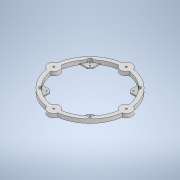
# Autodesk Inventor part: RL_spider_center_bottom_vt
Saved by Autodesk Inventor 2022 (Build 260153000, 153)
## iProperties
Created: 2021-08-09
Part Number: RL_spider_center_bottom_vt
Material: Generic
Document SubType Name: Modeling
Designer: james
Density: 1 g/cm^3
Appearance: Default
Author: james
Autodesk Inventor part; units mm, degrees
ref_plane "YZ Plane" through (0, 0, 0) normal (1, 0, 0) x (0, 1, 0)
ref_plane "XZ Plane" through (0, 0, 0) normal (0, 1, 0) x (-1, 0, 0)
ref_plane "XY Plane" through (0, 0, 0) normal (0, 0, 1) x (1, 0, 0)
sketch "Sketch1" plane through (0, 0, 0) normal (0, 1, 0) x (-1, 0, 0)
  circle A0 centre (0, 0) radius 100
  dimension "d0" = 200
  constraints: 1 centre point, 1 coincident
  measures "d0" diameter of A0
extrude "Extrusion1" add sketch "Sketch1" along normal blind 10
sketch "Sketch15" plane through (0, 10, 0) normal (0, 1, 0) x (1, 0, 0)
  circle A0 centre (0, 0) radius 90
  dimension "d139" = 180
  constraints: 1 centre point, 1 coincident
  measures "d139" diameter of A0
extrude "Extrusion13" cut sketch "Sketch15" against normal blind 20
sketch "Sketch19" plane through (0, 0, 0) normal (0, -1, 0) x (1, 0, 0)
  arc A0 (90, 0) -> (90, 0) centre (0, 0) ccw
  line L0 (49.497475, -56.568542) -> (56.568542, -49.497475)
  line L1 (0, 0) -> (53.033009, -53.033009)
  line L2 (0, 0) -> (1.922714, 0)
  line L3 (53.033009, -53.033009) -> (70.710678, -70.710678)
  circle A1 centre (0, 0) radius 100
  line L4 (49.497475, -56.568542) -> (49.497475, -75.166482)
  line L5 (56.568542, -49.497475) -> (75.166482, -49.497475)
  circle A2 centre (63.993164, -63.993164) radius 1.75
  circle A3 centre (56.922096, -56.922096) radius 1.75
  circle A4 centre (0, 0) radius 90
  point P0 (62.4461, -64.811146)
  point P1 (64.811146, -62.4461)
  dimension "d162" = 45
  dimension "d164" = 25
  dimension "d165" = 135
  dimension "d166" = 135
  dimension "d167" = 3.5
  dimension "d168" = 3.5
  dimension "d169" = 9.5
  dimension "d170" = 19.5
  dimension "d181" = 10
  constraints: 12 end point, 3 centre point, 2 point on circle, 2 point on line, 1 coincident, 1 horizontal, 1 midpoint, 1 perpendicular, 2 other
  measures "d162" angle of L1 L2
  measures "d164" distance from line of L3.end L0
  measures "d165" angle of L5 L0
  measures "d166" angle of L4 L0
  measures "d167" diameter of A3
  measures "d168" diameter of A2
  measures "d169" distance of L3.end A2.centre
  measures "d170" distance of L3.end A3.centre
  measures "d181" distance of L0.start L0.end
extrude "Extrusion16" add sketch "Sketch19" against normal blind 10 contours L4 L0 L3 A3 A2 A0 | A0 A2 L3 A3 L0 L5 | A2 L3 A0 | A0 L3 A2 | A2 L3 A0 | A0 L3 A2 | A3 L3 | L3 A3
sketch "Sketch20" plane through (0, 10, 0) normal (0, 1, 0) x (1, 0, 0)
  line L0 (49.497475, 56.568542) -> (56.568542, 49.497475)
  line L1 (53.033009, 53.033009) -> (70.710678, 70.710678)
  circle A0 centre (0, 0) radius 100
  circle A1 centre (63.993164, 63.993164) radius 1.75
  circle A2 centre (56.922096, 56.922096) radius 1.75
  dimension "d174" = 19.5
  dimension "d175" = 9.5
  dimension "d176" = 3.5
  dimension "d177" = 3.5
  constraints: 2 centre point, 2 end point, 2 point on line, 1 midpoint, 1 perpendicular, 2 other
  measures "d174" distance of A2.centre L1.end
  measures "d175" distance of A1.centre L1.end
  measures "d176" diameter of A1
  measures "d177" diameter of A2
extrude "Extrusion17" cut sketch "Sketch20" against normal blind 10 contours A2 L1 | L1 A2 | A1 L1 | L1 A1
sketch "Sketch21" plane through (0, 10, 0) normal (0, 1, 0) x (1, 0, 0)
  circle A0 centre (63.993164, 63.993164) radius 1.75
  arc A1 (67.528698, 60.45763) -> (60.45763, 67.528698) centre (63.993164, 63.993164) ccw
  line L0 (49.497475, 56.568542) -> (56.568542, 49.497475)
  line L1 (49.497475, 56.568542) -> (60.45763, 67.528698)
  line L2 (56.568542, 49.497475) -> (67.528698, 60.45763)
  arc A2 (49.497475, 75.166482) -> (75.166482, 49.497475) centre (0, 0) ccw
  arc A3 (75.166482, 49.497475) -> (49.497475, 75.166482) centre (0, 0) ccw
  line L3 (49.497475, 75.166482) -> (49.497475, 56.568542)
  line L4 (49.497475, 75.166482) -> (49.497475, 56.568542)
  line L5 (49.497475, 56.568542) -> (56.568542, 49.497475)
  line L6 (75.166482, 49.497475) -> (56.568542, 49.497475)
  line L7 (75.166482, 49.497475) -> (56.568542, 49.497475)
  point P0 (67.076859, 60.005791)
  point P1 (60.005791, 67.076859)
  point P2 (64.811146, 62.4461)
  point P3 (62.4461, 64.811146)
  dimension "d180" = 10
  constraints: 10 end point, 4 point on circle, 3 collinear, 2 centre point, 2 coincident, 2 perpendicular, 2 point on line, 2 tangent
  measures "d180" diameter of A1
extrude "Extrusion18" cut sketch "Sketch21" against normal blind 7 contours A0 A3 | A0 A3 L1 A1 L2 | A3 A0 | A0 A3 L2 L0 L1 | L1 L3 A3 | A3 L6 L2
fillet "Fillet1" radius 2 4 edges at (49.4975, 1.5, -56.5685) (56.5685, 1.5, -49.4975) (49.4975, 1.5, -75.1665) (75.1665, 1.5, -49.4975)
pattern_circular "Circular Pattern5" count 4 over 360 about axis through (0, -10, 0) along (0, 1, 0) of "Extrusion16", "Extrusion17", "Extrusion18", "Fillet1"
sketch "Sketch23" plane through (0, 10, 0) normal (0, 1, 0) x (1, 0, 0)
  circle A0 centre (-95, 0) radius 15
  arc A1 (-67.076859, 60.005791) -> (-67.076859, -60.005791) centre (0, 0) ccw
  circle A2 centre (0, -95) radius 15
  circle A3 centre (95, 0) radius 15
  circle A4 centre (0, 95) radius 15
  dimension "d210" = 95
  dimension "d211" = 30
  dimension "d214" = 360
  constraints: 4 centre point, 9 other
  measures "d210" distance of A1.centre A0.centre
  measures "d211" diameter of A0
extrude "Extrusion20" add sketch "Sketch23" against normal blind 10
sketch "Sketch22" plane through (0, 10, 0) normal (0, 1, 0) x (1, 0, 0)
  circle A0 centre (0, 95) radius 2.2
  circle A1 centre (-95, 0) radius 2.2
  circle A2 centre (0, -95) radius 2.2
  circle A3 centre (95, 0) radius 2.2
  point P0 (0, 0)
  dimension "d194" = 4.4
  dimension "d195" = 95
  dimension "d198" = 360
  constraints: 4 centre point, 9 other
  measures "d194" diameter of A0
  measures "d195" distance of point (0, 0) A0.centre
extrude "Extrusion21" cut sketch "Sketch22" against normal blind 10
body "Solid1"
